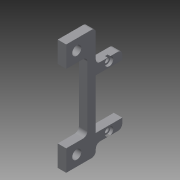
# Autodesk Inventor part: LongAxisServoSupport
Saved by Autodesk Inventor 2014 SP1 (Build 180222100, 222)
## iProperties
Created: 2017-05-14
Part Number: LongAxisServoSupport
Material: Generic
Document SubType Name: Modeling
Designer: danielsikar
Density: 1 g/cm^3
Appearance: Default
Author: danielsikar
Autodesk Inventor part; units mm, degrees
ref_plane "YZ Plane" through (0, 0, 0) normal (1, 0, 0) x (0, 1, 0)
ref_plane "XZ Plane" through (0, 0, 0) normal (0, 1, 0) x (-1, 0, 0)
ref_plane "Work Plane1" through (-18.8, 2.75, 32.2) normal (1, 0, 0) x (0, 0, -1)
sketch "Sketch1" plane through (-18.8, 2.75, 32.2) normal (1, 0, 0) x (0, 0, -1)
  line L0 (3.7, -5.65) -> (4.8, -5.65) projected
  line L1 (4.8, 0) -> (4.8, -5.65) projected
  line L2 (0, 0) -> (4.8, 0) projected
  line L3 (0, -12.5) -> (0, 0) projected
  line L4 (0, -12.5) -> (4.8, -12.5) projected
  line L5 (4.8, -6.85) -> (4.8, -12.5) projected
  line L6 (4.8, -6.85) -> (3.7, -6.85) projected
  arc A0 (3.7, -5.65) -> (3.7, -6.85) centre (2.9, -6.25) ccw projected
  line L7 (-26.5, -6.85) -> (-27.6, -6.85) projected
  line L8 (-27.6, -6.85) -> (-27.6, -12.5) projected
  line L9 (-22.8, -12.5) -> (-27.6, -12.5) projected
  line L10 (-22.8, 0) -> (-22.8, -12.5) projected
  line L11 (-22.8, 0) -> (-27.6, 0) projected
  line L12 (-27.6, 0) -> (-27.6, -5.65) projected
  line L13 (-27.6, -5.65) -> (-26.5, -5.65) projected
  arc A1 (-26.5, -6.85) -> (-26.5, -5.65) centre (-25.7, -6.25) ccw projected
  circle A2 centre (-25.7, -6.25) radius 1
  circle A3 centre (2.9, -6.25) radius 1
  line L14 (4.8, -5.25) -> (4.8, -7.1035)
  line L15 (-27.6, -4.6232) -> (-27.6, -7.8013)
  point P0 (32.2, -2.75)
  constraints: 4 end point, 4 point on line, 2 centre point, 2 coincident, 2 concentric
extrude "Extrusion1" add sketch "Sketch1" along normal blind 4 contours A0 L6 L5 L4 L3 L2 L1 L0 | A1 L13 L12 L11 L10 L9 L8 L7
sketch "Sketch2" plane through (-18.8, -2.9, 58.7) normal (0, -1, 0) x (1, 0, 0)
  line L0 (0, 1.1) -> (0, 0) projected
  line L1 (0, 0) -> (4, 0) projected
  line L2 (4, 1.1) -> (4, 0) projected
  line L3 (0, 1.1) -> (4, 1.1) projected
  point P0 (18.8, -58.7)
extrude "Extrusion2" add sketch "Sketch2" along normal blind 2
sketch "Sketch3" plane through (-14.8, 2.75, 32.2) normal (1, 0, 0) x (0, 0, -1)
  arc A0 (-26.5, -6.85) -> (-26.5, -5.65) centre (-25.7, -6.25) ccw projected
  line L0 (-26.5, -5.65) -> (-26.5, -6.85) projected
  circle A1 centre (-25.7, -6.25) radius 1
  point P0 (32.2, -2.75)
  constraints: 1 centre point, 1 coincident, 1 concentric
extrude "Extrusion3" cut sketch "Sketch3" against normal blind 4 contours A1 L0
sketch "Sketch4" plane through (-18.8, -2.9, 27.4) normal (0, -1, 0) x (1, 0, 0)
  line L0 (0, 1.1) -> (0, 0) projected
  line L1 (0, 0) -> (4, 0) projected
  line L2 (4, 1.1) -> (4, 0) projected
  line L3 (0, 1.1) -> (4, 1.1) projected
  point P0 (18.8, -27.4)
extrude "Extrusion4" add sketch "Sketch4" along normal blind 4
sketch "Sketch5" plane through (-14.8, 2.75, 32.2) normal (1, 0, 0) x (0, 0, -1)
  arc A0 (3.7, -5.65) -> (3.7, -6.85) centre (2.9, -6.25) ccw projected
  line L0 (3.7, -5.65) -> (3.7, -6.85) projected
  circle A1 centre (2.9, -6.25) radius 1
  point P0 (32.2, -2.75)
  constraints: 1 centre point, 1 coincident, 1 concentric
extrude "Extrusion5" cut sketch "Sketch5" against normal blind 4 contours A1 L0
sketch "Sketch6" plane through (-18.8, -9.75, 55) normal (0, 0, -1) x (-1, 0, 0)
  line L0 (0, 0) -> (0, 12.5) projected
  line L1 (0, 12.5) -> (-4, 12.5) projected
  line L2 (-4, 0) -> (-4, 12.5) projected
  line L3 (0, 0) -> (-4, 0) projected
  point P0 (-18.8, 9.75)
extrude "Extrusion6" cut sketch "Sketch6" against normal blind 0.4
sketch "Sketch7" plane through (-18.8, -9.75, 32.2) normal (0, 0, 1) x (1, 0, 0)
  line L0 (0, 12.5) -> (0, 0) projected
  line L1 (0, 0) -> (4, 0) projected
  line L2 (4, 12.5) -> (4, 0) projected
  line L3 (0, 12.5) -> (4, 12.5) projected
  point P0 (18.8, 9.75)
extrude "Extrusion7" cut sketch "Sketch7" against normal blind 0.4
sketch "Sketch8" plane through (-18.8, -9.75, 59.8) normal (0, -1, 0) x (1, 0, 0)
  line L0 (0, -32.4) -> (4, -32.4) projected
  line L1 (4, -28) -> (4, -32.4) projected
  line L2 (0, 0) -> (4, 0)
  line L3 (4, 0) -> (4, -32.4)
  line L4 (4, -32.4) -> (0, -32.4)
  line L5 (0, -32.4) -> (0, 0)
  point P0 (18.8, -59.8)
  constraints: 8 end point, 2 parallel, 1 horizontal, 1 perpendicular
extrude "Extrusion8" add sketch "Sketch8" along normal blind 4
fillet "Fillet1" radius 2 2 edges at (-16.8, 2.75, 59.8) (-16.8, 2.75, 27.4)
sketch "Sketch9" plane through (-18.8, -13.75, 59.8) normal (0, 0, 1) x (1, 0, 0)
  line L0 (4, 14.5) -> (4, 0) projected
  line L1 (0, 0) -> (4, 0)
  line L2 (4, 0) -> (4, 4)
  line L3 (4, 4) -> (0, 4)
  line L4 (0, 4) -> (0, 0)
  point P0 (18.8, 13.75)
  dimension "d17" = 4
  constraints: 8 end point, 2 parallel, 1 horizontal, 1 perpendicular, 1 point on line
  measures "d17" distance of L2.end L1.end
extrude "Extrusion9" add sketch "Sketch9" along normal blind 10
sketch "Sketch10" plane through (-14.8, -13.75, 27.4) normal (0, 0, -1) x (-1, 0, 0)
  line L0 (0, 0) -> (4, 0)
  line L1 (4, 0) -> (4, 4)
  line L2 (4, 4) -> (0, 4)
  line L3 (0, 4) -> (0, 0)
  point P0 (-14.8, 13.75)
  dimension "d20" = 4
  dimension "d21" = 4
  constraints: 8 end point, 2 parallel, 1 horizontal, 1 perpendicular
  measures "d20" distance of L2.end L1.end
  measures "d21" distance of L1.end L0.end
extrude "Extrusion10" add sketch "Sketch10" along normal blind 10
sketch "Sketch15" plane through (-14.8, 2.75, 32.2) normal (1, 0, 0) x (0, 0, -1)
  circle A0 centre (-25.7, -6.25) radius 1 projected
  circle A1 centre (-25.7, -6.25) radius 1.25
  point P0 (32.2, -2.75)
  dimension "d42" = 2.5
  constraints: 1 centre point, 1 coincident
  measures "d42" diameter of A1
extrude "Extrusion15" cut sketch "Sketch15" against normal blind 5
sketch "Sketch16" plane through (-14.8, 2.75, 32.2) normal (1, 0, 0) x (0, 0, -1)
  circle A0 centre (2.9, -6.25) radius 1 projected
  circle A1 centre (2.9, -6.25) radius 1.25
  point P0 (32.2, -2.75)
  dimension "d45" = 2.5
  constraints: 1 centre point, 1 coincident
  measures "d45" diameter of A1
extrude "Extrusion16" cut sketch "Sketch16" against normal blind 5
sketch "Sketch17" plane through (-14.8, 2.75, 32.2) normal (1, 0, 0) x (0, 0, -1)
  circle A0 centre (-25.7, -6.25) radius 1.25 projected
  circle A1 centre (-25.7, -6.25) radius 2
  point P0 (32.2, -2.75)
  dimension "d48" = 4
  constraints: 1 centre point, 1 coincident
  measures "d48" diameter of A1
extrude "Extrusion17" cut sketch "Sketch17" against normal blind 1.3
sketch "Sketch18" plane through (-14.8, 2.75, 32.2) normal (1, 0, 0) x (0, 0, -1)
  circle A0 centre (2.9, -6.25) radius 1.25 projected
  circle A1 centre (2.9, -6.25) radius 2
  point P0 (32.2, -2.75)
  dimension "d51" = 4
  constraints: 1 centre point, 1 coincident
  measures "d51" diameter of A1
extrude "Extrusion18" cut sketch "Sketch18" against normal blind 1.3
sketch "Sketch19" plane through (-14.8, -13.75, 17.4) normal (0, 0, -1) x (-1, 0, 0)
  line L0 (0, 0) -> (4, 0) projected
  line L1 (4, 0) -> (4, 4) projected
  line L2 (4, 4) -> (0, 4) projected
  line L3 (0, 4) -> (0, 0) projected
  point P0 (-14.8, 13.75)
extrude "Extrusion19" cut sketch "Sketch19" against normal blind 5.1
sketch "Sketch20" plane through (-18.8, -13.75, 69.8) normal (0, 0, 1) x (1, 0, 0)
  line L0 (0, 0) -> (4, 0) projected
  line L1 (4, 0) -> (4, 4) projected
  line L2 (4, 4) -> (0, 4) projected
  line L3 (0, 4) -> (0, 0) projected
  point P0 (18.8, 13.75)
extrude "Extrusion20" add sketch "Sketch20" along normal blind 5.2
sketch "Sketch21" plane through (-18.8, -13.75, 59.8) normal (0, -1, 0) x (1, 0, 0)
  line L0 (0, -37.3) -> (4, -37.3) projected
  line L1 (4, 15.2) -> (4, -37.3) projected
  line L2 (0, -37.3) -> (4, -37.3)
  line L3 (4, -37.3) -> (4, -27.3)
  line L4 (4, -27.3) -> (0, -27.3)
  line L5 (0, -27.3) -> (0, -37.3)
  line L6 (0, 15.2) -> (4, 15.2)
  line L7 (4, 15.2) -> (4, 5.2)
  line L8 (4, 5.2) -> (0, 5.2)
  line L9 (0, 5.2) -> (0, 15.2)
  point P0 (18.8, -59.8)
  dimension "d58" = 10
  dimension "d59" = 10
  constraints: 16 end point, 4 parallel, 2 horizontal, 2 perpendicular, 2 point on line
  measures "d58" distance of L3.end L2.end
  measures "d59" distance of L6.end L7.end
extrude "Extrusion21" add sketch "Sketch21" along normal blind 6
sketch "Sketch22" plane through (-18.8, 2.75, 32.2) normal (-1, 0, 0) x (0, 0, 1)
  circle A0 centre (37.8, -21.5) radius 2.15
  line L0 (27.6, -12.5) -> (42.8, -12.5) projected
  point P0 (-32.2, -2.75)
  dimension "d62" = 4.3
  dimension "d74" = 9
  constraints: 1 centre point
  measures "d62" diameter of A0
  measures "d74" distance from line of A0.centre L0
extrude "Extrusion22" cut sketch "Sketch22" against normal blind 6
sketch "Sketch23" plane through (-18.8, 2.75, 32.2) normal (-1, 0, 0) x (0, 0, 1)
  line L0 (0.3, -16.5) -> (0.3, -22.5) projected
  circle A0 centre (-4.7, -21.5) radius 2.15
  line L1 (-4.8, -12.5) -> (-9.7, -12.5) projected
  point P0 (-32.2, -2.75)
  dimension "d65" = 4.3
  dimension "d66" = 5
  dimension "d75" = 9
  constraints: 1 centre point
  measures "d65" diameter of A0
  measures "d66" distance from line of L0 A0.centre
  measures "d75" distance from line of A0.centre L1
extrude "Extrusion23" cut sketch "Sketch23" against normal blind 6
fillet "Fillet5" radius 2 6 edges at (-16.8, -9.75, 75) (-16.8, -9.75, 59.8) (-16.8, -13.75, 65) (-16.8, -9.75, 27.4) (-16.8, -9.75, 22.5) (-16.8, -13.75, 32.5)
sketch "Sketch24" plane through (-18.8, -19.75, 59.8) normal (0, -1, 0) x (1, 0, 0)
  line L0 (4, 5.2) -> (4, 15.2) projected
  line L1 (4, 15.2) -> (0, 15.2) projected
  line L2 (0, 15.2) -> (0, 5.2) projected
  line L3 (0, 5.2) -> (4, 5.2) projected
  point P0 (18.8, -59.8)
extrude "Extrusion24" add sketch "Sketch24" along normal blind 4
sketch "Sketch25" plane through (-18.8, -19.75, 59.8) normal (0, -1, 0) x (1, 0, 0)
  line L0 (0, -37.3) -> (4, -37.3) projected
  line L1 (4, -37.3) -> (4, -27.3) projected
  line L2 (4, -27.3) -> (0, -27.3) projected
  line L3 (0, -27.3) -> (0, -37.3) projected
  point P0 (18.8, -59.8)
extrude "Extrusion25" add sketch "Sketch25" along normal blind 4
sketch "Sketch26" plane through (-18.8, 2.75, 32.2) normal (-1, 0, 0) x (0, 0, 1)
  line L0 (-2.7967, -22.5) -> (-6.6033, -22.5) projected
  arc A0 (-2.7967, -22.5) -> (-6.6033, -22.5) centre (-4.7, -21.5) ccw projected
  circle A1 centre (-4.7, -21.5) radius 2.15
  point P0 (-32.2, -2.75)
  dimension "d76" = 4.3
  constraints: 1 centre point, 1 coincident
  measures "d76" diameter of A1
extrude "Extrusion26" cut sketch "Sketch26" against normal blind 4 contours A1 L0
sketch "Sketch27" plane through (-18.8, 2.75, 32.2) normal (-1, 0, 0) x (0, 0, 1)
  arc A0 (39.7033, -22.5) -> (35.8967, -22.5) centre (37.8, -21.5) ccw projected
  line L0 (39.7033, -22.5) -> (35.8967, -22.5) projected
  circle A1 centre (37.8, -21.5) radius 2.15
  point P0 (-32.2, -2.75)
  dimension "d79" = 4.3
  constraints: 1 centre point, 1 coincident
  measures "d79" diameter of A1
extrude "Extrusion27" cut sketch "Sketch27" against normal blind 4 contours A1 L0
body "Solid1"
